Autodesk Fusion 360 part; units mm, degrees
note: some values were not read from the file. Chosen so that the rebuilt part matches the saved one: which pieces of a blend or face edit are solid. Set by a fixed rule: which sketch regions a step uses.
(part 2 of 2)
  line L392 (-39.9447, 99.1082) -> (-40.4511, 101.9789)
  line L393 (-40.4511, 101.9789) -> (-40.8173, 104.0543)
  line L394 (-40.8173, 104.0543) -> (-41.1737, 106.0754)
  line L395 (-41.1737, 106.0754) -> (-42.1677, 111.7124)
  line L396 (-42.1677, 111.7124) -> (-51.7977, 110.0143)
  line L397 (-51.7977, 110.0143) -> (-57.5307, 109.0036)
  line L398 (-57.5307, 109.0036) -> (-57.0143, 106.0757)
  line L399 (-57.0143, 106.0757) -> (-56.9434, 105.6722)
  line L400 (-22.1028, 107.3526) -> (-22.6759, 110.6014)
  line L401 (-22.6759, 110.6014) -> (-23.3222, 114.2669)
  line L402 (-23.3222, 114.2669) -> (-24.0445, 118.3627)
  line L403 (-24.0445, 118.3627) -> (-24.3258, 119.9557)
  line L404 (-24.3258, 119.9557) -> (-27.2217, 119.4446)
  line L405 (-27.2217, 119.4446) -> (-35.4137, 118.0002)
  line L406 (-35.4137, 118.0002) -> (-39.6875, 117.2461)
  line L407 (-39.6875, 117.2461) -> (-39.1623, 114.2664)
  line L408 (-39.1623, 114.2664) -> (-38.816, 112.3021)
  line L409 (-38.816, 112.3021) -> (-37.7177, 106.0746)
  line L410 (-37.7177, 106.0746) -> (-37.4658, 104.6443)
  line L411 (-37.4658, 104.6443) -> (-35.4137, 105.006)
  line L412 (-35.4137, 105.006) -> (-29.3531, 106.0746)
  line L413 (-29.3531, 106.0746) -> (-22.1028, 107.3526)
  line L414 (-85.4379, 28.9057) -> (-100.801, 26.198)
  line L415 (-100.801, 26.198) -> (-98.9954, 15.9628)
  line L416 (-98.9954, 15.9628) -> (-98.5779, 13.5969)
  line L417 (-98.5779, 13.5969) -> (-85.1554, 15.9628)
  line L418 (-85.1554, 15.9628) -> (-84.5661, 16.0668)
  line L419 (-84.5661, 16.0668) -> (-83.2149, 16.3049)
  line L420 (-83.2149, 16.3049) -> (-84.5661, 23.9628)
  line L421 (-84.5661, 23.9628) -> (-85.4379, 28.9057)
  line L422 (-105.1938, 50.9886) -> (-100.9499, 51.7366)
  line L423 (-100.9499, 51.7366) -> (-92.7579, 53.1807)
  line L424 (-92.7579, 53.1807) -> (-89.8308, 53.6967)
  line L425 (-89.8308, 53.6967) -> (-90.3997, 56.9225)
  line L426 (-90.3997, 56.9225) -> (-91.8451, 65.1145)
  line L427 (-91.8451, 65.1145) -> (-92.0538, 66.2977)
  line L428 (-92.0538, 66.2977) -> (-92.7576, 66.1736)
  line L429 (-92.7576, 66.1736) -> (-98.7671, 65.1145)
  line L430 (-98.7671, 65.1145) -> (-100.9497, 64.73)
  line L431 (-100.9497, 64.73) -> (-107.4155, 63.5905)
  line L432 (-107.4155, 63.5905) -> (-107.4018, 63.513)
  line L433 (-107.4018, 63.513) -> (-106.2397, 56.9225)
  line L434 (-106.2397, 56.9225) -> (-105.1938, 50.9886)
  line L435 (-47.6311, 52.8267) -> (-46.9085, 48.731)
  line L436 (-46.9085, 48.731) -> (-46.5989, 46.976)
  line L437 (-46.5989, 46.976) -> (-45.4636, 40.5389)
  line L438 (-45.4636, 40.5389) -> (-45.4099, 40.2339)
  line L439 (-45.4099, 40.2339) -> (-43.6795, 40.5389)
  line L440 (-43.6795, 40.5389) -> (-35.4139, 41.996)
  line L441 (-35.4139, 41.996) -> (-30.0471, 42.9419)
  line L442 (-30.0471, 42.9419) -> (-31.0682, 48.731)
  line L443 (-31.0682, 48.731) -> (-32.2699, 55.545)
  line L444 (-32.2699, 55.545) -> (-35.4139, 54.9907)
  line L445 (-35.4139, 54.9907) -> (-43.606, 53.5466)
  line L446 (-43.606, 53.5466) -> (-47.6332, 52.8368)
  line L447 (-47.6332, 52.8368) -> (-47.6311, 52.8267)
  line L448 (-44.1788, 34.1749) -> (-43.856, 32.3469)
  line L449 (-43.856, 32.3469) -> (-42.4101, 24.1549)
  line L450 (-42.4101, 24.1549) -> (-41.9545, 21.5739)
  line L451 (-41.9545, 21.5739) -> (-35.4134, 22.7267)
  line L452 (-35.4134, 22.7267) -> (-27.3129, 24.1546)
  line L453 (-27.3129, 24.1546) -> (-26.5925, 24.2813)
  line L454 (-26.5925, 24.2813) -> (-28.0151, 32.3464)
  line L455 (-28.0151, 32.3464) -> (-28.8152, 36.8832)
  line L456 (-28.8152, 36.8832) -> (-35.4134, 35.7198)
  line L457 (-35.4134, 35.7198) -> (-43.6055, 34.2754)
  line L458 (-43.6055, 34.2754) -> (-44.1788, 34.1749)
  line L459 (-76.3738, 14.4656) -> (-68.1818, 15.9097)
  line L460 (-68.1818, 15.9097) -> (-67.881, 15.9626)
  line L461 (-67.881, 15.9626) -> (-63.9839, 16.6497)
  line L462 (-63.9839, 16.6497) -> (-65.3079, 24.1546)
  line L463 (-65.3079, 24.1546) -> (-66.0299, 28.2506)
  line L464 (-66.0299, 28.2506) -> (-66.2067, 29.2515)
  line L465 (-66.2067, 29.2515) -> (-68.1818, 28.9033)
  line L466 (-68.1818, 28.9033) -> (-81.57, 26.5435)
  line L467 (-81.57, 26.5435) -> (-79.7026, 15.9626)
  line L468 (-79.7026, 15.9626) -> (-79.3459, 13.9414)
  line L469 (-79.3459, 13.9414) -> (-76.3738, 14.4656)
  line L470 (-17.1048, 98.5898) -> (-2.6458, 101.138)
  line L471 (-2.6458, 101.138) -> (-1.7428, 101.2973)
  line L472 (-1.7428, 101.2973) -> (-2.6458, 106.4194)
  line L473 (-2.6458, 106.4194) -> (-3.9648, 113.901)
  line L474 (-3.9648, 113.901) -> (-19.0296, 111.2443)
  line L475 (-19.0296, 111.2443) -> (-19.3275, 111.1922)
  line L476 (-19.3275, 111.1922) -> (-19.0296, 109.5023)
  line L477 (-19.0296, 109.5023) -> (-17.1048, 98.5898)
  line L478 (-27.2217, 48.5214) -> (-26.035, 48.7307)
  line L479 (-26.035, 48.7307) -> (-19.0296, 49.966)
  line L480 (-19.0296, 49.966) -> (-12.1245, 51.1839)
  line L481 (-12.1245, 51.1839) -> (-13.1366, 56.9227)
  line L482 (-13.1366, 56.9227) -> (-14.3465, 63.7855)
  line L483 (-14.3465, 63.7855) -> (-19.0294, 62.9603)
  line L484 (-19.0294, 62.9603) -> (-27.2214, 61.5162)
  line L485 (-27.2214, 61.5162) -> (-29.7093, 61.0777)
  line L486 (-29.7093, 61.0777) -> (-29.699, 61.0187)
  line L487 (-29.699, 61.0187) -> (-28.9766, 56.9227)
  line L488 (-28.9766, 56.9227) -> (-27.5315, 48.7307)
  line L489 (-27.5315, 48.7307) -> (-27.4865, 48.4746)
  line L490 (-27.4865, 48.4746) -> (-27.2217, 48.5214)
  line L491 (-59.7657, 12.3216) -> (-51.7977, 13.7266)
  line L492 (-51.7977, 13.7266) -> (-44.4037, 15.0299)
  line L493 (-44.4037, 15.0299) -> (-44.5685, 15.9628)
  line L494 (-44.5685, 15.9628) -> (-46.0134, 24.1549)
  line L495 (-46.0134, 24.1549) -> (-46.6267, 27.632)
  line L496 (-46.6267, 27.632) -> (-51.7977, 26.7203)
  line L497 (-51.7977, 26.7203) -> (-59.9898, 25.2756)
  line L498 (-59.9898, 25.2756) -> (-61.9898, 24.9232)
  line L499 (-61.9898, 24.9232) -> (-61.8543, 24.1551)
  line L500 (-61.8543, 24.1551) -> (-60.4083, 15.9631)
  line L501 (-60.4083, 15.9631) -> (-59.9898, 13.5911)
  line L502 (-59.9898, 13.5911) -> (-59.7657, 12.3216)
  line L503 (-117.334, 10.2986) -> (-109.1417, 11.7422)
  line L504 (-109.1417, 11.7422) -> (-108.4355, 11.8668)
  line L505 (-108.4355, 11.8668) -> (-102.0228, 12.9969)
  line L506 (-102.0228, 12.9969) -> (-102.5459, 15.9628)
  line L507 (-102.5459, 15.9628) -> (-103.9902, 24.1549)
  line L508 (-103.9902, 24.1549) -> (-104.2448, 25.599)
  line L509 (-104.2448, 25.599) -> (-109.1419, 24.7356)
  line L510 (-109.1419, 24.7356) -> (-112.4368, 24.1549)
  line L511 (-112.4368, 24.1549) -> (-117.3342, 23.2915)
  line L512 (-117.3342, 23.2915) -> (-119.6081, 22.8907)
  line L513 (-119.6081, 22.8907) -> (-118.386, 15.9626)
  line L514 (-118.386, 15.9626) -> (-117.385, 10.2896)
  line L515 (-117.385, 10.2896) -> (-117.334, 10.2986)
  line L516 (-72.925, 87.1937) -> (-68.1818, 88.0298)
  line L517 (-68.1818, 88.0298) -> (-58.7589, 89.6906)
  line L518 (-58.7589, 89.6906) -> (-57.562, 89.902)
  line L519 (-57.562, 89.902) -> (-58.2472, 93.7866)
  line L520 (-58.2472, 93.7866) -> (-58.9695, 97.8829)
  line L521 (-58.9695, 97.8829) -> (-59.7847, 102.5059)
  line L522 (-59.7847, 102.5059) -> (-68.1818, 101.0259)
  line L523 (-68.1818, 101.0259) -> (-75.1478, 99.7974)
  line L524 (-75.1478, 99.7974) -> (-74.8101, 97.8829)
  line L525 (-74.8101, 97.8829) -> (-73.3653, 89.6906)
  line L526 (-73.3653, 89.6906) -> (-72.925, 87.1937)
  line L527 (-84.5661, 90.283) -> (-77.1416, 91.5919)
  line L528 (-77.1416, 91.5919) -> (-78.2505, 97.8829)
  line L529 (-78.2505, 97.8829) -> (-79.3636, 104.1966)
  line L530 (-79.3636, 104.1966) -> (-84.5659, 103.2793)
  line L531 (-84.5659, 103.2793) -> (-94.7266, 101.4868)
  line L532 (-94.7266, 101.4868) -> (-94.0911, 97.8829)
  line L533 (-94.0911, 97.8829) -> (-92.646, 89.6906)
  line L534 (-92.646, 89.6906) -> (-92.5036, 88.8839)
  line L535 (-92.5036, 88.8839) -> (-87.9258, 89.6906)
  line L536 (-87.9258, 89.6906) -> (-84.5661, 90.283)
  line L537 (-117.334, 29.5698) -> (-109.1417, 31.0139)
  line L538 (-109.1417, 31.0139) -> (-105.2335, 31.7029)
  line L539 (-105.2335, 31.7029) -> (-105.3473, 32.3469)
  line L540 (-105.3473, 32.3469) -> (-106.7922, 40.5389)
  line L541 (-106.7922, 40.5389) -> (-107.4568, 44.3058)
  line L542 (-107.4568, 44.3058) -> (-109.1417, 44.0087)
  line L543 (-109.1417, 44.0087) -> (-117.334, 42.5643)
  line L544 (-117.334, 42.5643) -> (-122.8199, 41.597)
  line L545 (-122.8199, 41.597) -> (-122.6331, 40.5389)
  line L546 (-122.6331, 40.5389) -> (-121.1879, 32.3469)
  line L547 (-121.1879, 32.3469) -> (-120.5968, 28.9949)
  line L548 (-120.5968, 28.9949) -> (-117.334, 29.5698)
  line L549 (-89.2709, 70.0887) -> (-84.5661, 70.9187)
  line L550 (-84.5661, 70.9187) -> (-76.3738, 72.363)
  line L551 (-76.3738, 72.363) -> (-73.9079, 72.7977)
  line L552 (-73.9079, 72.7977) -> (-73.9979, 73.3073)
  line L553 (-73.9979, 73.3073) -> (-75.4428, 81.4991)
  line L554 (-75.4428, 81.4991) -> (-75.8899, 84.0354)
  line L555 (-75.8899, 84.0354) -> (-76.1309, 85.4012)
  line L556 (-76.1309, 85.4012) -> (-76.3738, 85.3583)
  line L557 (-76.3738, 85.3583) -> (-84.5661, 83.9134)
  line L558 (-84.5661, 83.9134) -> (-91.4143, 82.7061)
  line L559 (-91.4143, 82.7061) -> (-91.494, 82.6916)
  line L560 (-91.494, 82.6916) -> (-91.2836, 81.4988)
  line L561 (-91.2836, 81.4988) -> (-89.8385, 73.3071)
  line L562 (-89.8385, 73.3071) -> (-89.2709, 70.0887)
  line L563 (-116.8487, 97.8829) -> (-117.3057, 100.4729)
  line L564 (-117.3057, 100.4729) -> (-117.334, 100.4676)
  line L565 (-117.334, 100.4676) -> (-125.5257, 99.0232)
  line L566 (-125.5257, 99.0232) -> (-131.9937, 97.8826)
  line L567 (-131.9937, 97.8826) -> (-132.6687, 97.7633)
  line L568 (-132.6687, 97.7633) -> (-130.4459, 85.1604)
  line L569 (-130.4459, 85.1604) -> (-117.334, 87.4723)
  line L570 (-117.334, 87.4723) -> (-115.0829, 87.8692)
  line L571 (-115.0829, 87.8692) -> (-115.4038, 89.6903)
  line L572 (-115.4038, 89.6903) -> (-116.8487, 97.8829)
  line L573 (-65.2976, 43.6798) -> (-64.7435, 40.5387)
  line L574 (-64.7435, 40.5387) -> (-63.2987, 32.3466)
  line L575 (-63.2987, 32.3466) -> (-63.0746, 31.0756)
  line L576 (-63.0746, 31.0756) -> (-59.9895, 31.6196)
  line L577 (-59.9895, 31.6196) -> (-55.8665, 32.3466)
  line L578 (-55.8665, 32.3466) -> (-51.7975, 33.0642)
  line L579 (-51.7975, 33.0642) -> (-47.7115, 33.7849)
  line L580 (-47.7115, 33.7849) -> (-48.1804, 36.4427)
  line L581 (-48.1804, 36.4427) -> (-48.9027, 40.5387)
  line L582 (-48.9027, 40.5387) -> (-49.9343, 46.3875)
  line L583 (-49.9343, 46.3875) -> (-51.7972, 46.0592)
  line L584 (-51.7972, 46.0592) -> (-65.2976, 43.6798)
  line L585 (-110.7239, 82.346) -> (-110.7107, 82.2711)
  line L586 (-110.7107, 82.2711) -> (-110.5741, 81.4991)
  line L587 (-110.5741, 81.4991) -> (-109.13, 73.3073)
  line L588 (-109.13, 73.3073) -> (-108.5017, 69.7426)
  line L589 (-108.5017, 69.7426) -> (-100.9497, 71.0748)
  line L590 (-100.9497, 71.0748) -> (-93.1386, 72.4519)
  line L591 (-93.1386, 72.4519) -> (-93.2894, 73.307)
  line L592 (-93.2894, 73.307) -> (-94.7343, 81.4988)
  line L593 (-94.7343, 81.4988) -> (-95.3617, 85.0545)
  line L594 (-95.3617, 85.0545) -> (-100.9497, 84.069)
  line L595 (-100.9497, 84.069) -> (-109.1417, 82.6246)
  line L596 (-109.1417, 82.6246) -> (-110.7239, 82.346)
  line L597 (-51.0701, 52.8267) -> (-51.7927, 56.9227)
  line L598 (-51.7927, 56.9227) -> (-51.7977, 56.951)
  line L599 (-51.7977, 56.951) -> (-53.2376, 65.1145)
  line L600 (-53.2376, 65.1145) -> (-53.2429, 65.1423)
  line L601 (-53.2429, 65.1423) -> (-53.2585, 65.1396)
  line L602 (-53.2585, 65.1396) -> (-53.4016, 65.1142)
  line L603 (-53.4016, 65.1142) -> (-68.1818, 62.5078)
  line L604 (-68.1818, 62.5078) -> (-68.6059, 62.4332)
  line L605 (-68.6059, 62.4332) -> (-68.1818, 60.0297)
  line L606 (-68.1818, 60.0297) -> (-66.3826, 49.8322)
  line L607 (-66.3826, 49.8322) -> (-51.7977, 52.4031)
  line L608 (-51.7977, 52.4031) -> (-51.0199, 52.5404)
  line L609 (-51.0199, 52.5404) -> (-51.0701, 52.8267)
  line L610 (-114.0727, 81.6777) -> (-115.0874, 81.4988)
  line L611 (-115.0874, 81.4988) -> (-117.334, 81.1025)
  line L612 (-117.334, 81.1025) -> (-129.4347, 78.9678)
  line L613 (-129.4347, 78.9678) -> (-128.4367, 73.3071)
  line L614 (-128.4367, 73.3071) -> (-127.2127, 66.3649)
  line L615 (-127.2127, 66.3649) -> (-117.334, 68.1069)
  line L616 (-117.334, 68.1069) -> (-111.8494, 69.0737)
  line L617 (-111.8494, 69.0737) -> (-112.5961, 73.3071)
  line L618 (-112.5961, 73.3071) -> (-114.041, 81.4988)
  line L619 (-114.041, 81.4988) -> (-114.0727, 81.6777)
  line L620 (-11.0397, 45.0308) -> (-19.0296, 43.6219)
  line L621 (-19.0296, 43.6219) -> (-26.4014, 42.322)
  line L622 (-26.4014, 42.322) -> (-26.0871, 40.5389)
  line L623 (-26.0871, 40.5389) -> (-25.5442, 37.4608)
  line L624 (-25.5442, 37.4608) -> (-24.642, 32.3469)
  line L625 (-24.642, 32.3469) -> (-24.1787, 29.7209)
  line L626 (-24.1787, 29.7209) -> (-19.0296, 30.6287)
  line L627 (-19.0296, 30.6287) -> (-9.2818, 32.3469)
  line L628 (-9.2818, 32.3469) -> (-8.8164, 32.4292)
  line L629 (-8.8164, 32.4292) -> (-11.0397, 45.0308)
  line L630 (-52.0089, 77.6719) -> (-51.7977, 77.7092)
  line L631 (-51.7977, 77.7092) -> (-43.6057, 79.1541)
  line L632 (-43.6057, 79.1541) -> (-39.51, 79.8769)
  line L633 (-39.51, 79.8769) -> (-36.6458, 80.3817)
  line L634 (-36.6458, 80.3817) -> (-36.843, 81.4991)
  line L635 (-36.843, 81.4991) -> (-38.8689, 92.9841)
  line L636 (-38.8689, 92.9841) -> (-51.7977, 90.7052)
  line L637 (-51.7977, 90.7052) -> (-54.2316, 90.2758)
  line L638 (-54.2316, 90.2758) -> (-54.1285, 89.6908)
  line L639 (-54.1285, 89.6908) -> (-52.6836, 81.4991)
  line L640 (-52.6836, 81.4991) -> (-52.0089, 77.6719)
  line L641 (-15.4329, 69.94) -> (-17.472, 81.4991)
  line L642 (-17.472, 81.4991) -> (-17.6559, 82.541)
  line L643 (-17.6559, 82.541) -> (-19.0296, 82.2992)
  line L644 (-19.0296, 82.2992) -> (-23.5667, 81.4993)
  line L645 (-23.5667, 81.4993) -> (-27.2214, 80.8548)
  line L646 (-27.2214, 80.8548) -> (-33.0174, 79.8332)
  line L647 (-33.0174, 79.8332) -> (-32.5906, 77.4147)
  line L648 (-32.5906, 77.4147) -> (-32.5887, 77.4033)
  line L649 (-32.5887, 77.4033) -> (-32.4734, 76.7495)
  line L650 (-32.4734, 76.7495) -> (-32.2932, 75.7298)
  line L651 (-32.2932, 75.7298) -> (-32.227, 75.3546)
  line L652 (-32.227, 75.3546) -> (-31.8659, 73.3073)
  line L653 (-31.8659, 73.3073) -> (-30.7941, 67.2322)
  line L654 (-30.7941, 67.2322) -> (-19.0291, 69.306)
  line L655 (-19.0291, 69.306) -> (-15.4329, 69.94)
  line L656 (-71.1078, 56.9227) -> (-71.9749, 61.8395)
  line L657 (-71.9749, 61.8395) -> (-72.5533, 65.1148)
  line L658 (-72.5533, 65.1148) -> (-72.8231, 66.644)
  line L659 (-72.8231, 66.644) -> (-76.3738, 66.0178)
  line L660 (-76.3738, 66.0178) -> (-81.497, 65.1148)
  line L661 (-81.497, 65.1148) -> (-84.5661, 64.5737)
  line L662 (-84.5661, 64.5737) -> (-88.1859, 63.9358)
  line L663 (-88.1859, 63.9358) -> (-86.9487, 56.9227)
  line L664 (-86.9487, 56.9227) -> (-86.2264, 52.8267)
  line L665 (-86.2264, 52.8267) -> (-85.9631, 51.3347)
  line L666 (-85.9631, 51.3347) -> (-84.5664, 51.581)
  line L667 (-84.5664, 51.581) -> (-70.6004, 54.0427)
  line L668 (-70.6004, 54.0427) -> (-71.1078, 56.9227)
  line L669 (-110.7649, 62.9206) -> (-117.334, 61.7627)
  line L670 (-117.334, 61.7627) -> (-125.5257, 60.3189)
  line L671 (-125.5257, 60.3189) -> (-126.1277, 60.2128)
  line L672 (-126.1277, 60.2128) -> (-125.5474, 56.9227)
  line L673 (-125.5474, 56.9227) -> (-124.1026, 48.7307)
  line L674 (-124.1026, 48.7307) -> (-123.9046, 47.6107)
  line L675 (-123.9046, 47.6107) -> (-123.8814, 47.6149)
  line L676 (-123.8814, 47.6149) -> (-117.5531, 48.731)
  line L677 (-117.5531, 48.731) -> (-117.334, 48.7696)
  line L678 (-117.334, 48.7696) -> (-108.5419, 50.3198)
  line L679 (-108.5419, 50.3198) -> (-109.7068, 56.9227)
  line L680 (-109.7068, 56.9227) -> (-110.7649, 62.9206)
  line L681 (-50.8616, 71.5666) -> (-49.7234, 65.1148)
  line L682 (-49.7234, 65.1148) -> (-48.6386, 58.9658)
  line L683 (-48.6386, 58.9658) -> (-35.4137, 61.2979)
  line L684 (-35.4137, 61.2979) -> (-33.2766, 61.6746)
  line L685 (-33.2766, 61.6746) -> (-33.8831, 65.1148)
  line L686 (-33.8831, 65.1148) -> (-35.3269, 73.307)
  line L687 (-35.3269, 73.307) -> (-35.4137, 73.7989)
  line L688 (-35.4137, 73.7989) -> (-35.4976, 74.2754)
  line L689 (-35.4976, 74.2754) -> (-39.5097, 73.5685)
  line L690 (-39.5097, 73.5685) -> (-40.9932, 73.307)
  line L691 (-40.9932, 73.307) -> (-50.8616, 71.5666)
  circle A2 centre (-9.2275, 58.7363) radius 1.1
  circle A3 centre (-44.1849, 9.3587) radius 1.1
  circle A4 centre (-19.4818, 116.8758) radius 1.1
  circle A5 centre (-35.5447, 77.4392) radius 1.1
  circle A6 centre (-61.567, 107.9028) radius 1.1
  circle A7 centre (-85.9131, 48.171) radius 1.1
  circle A8 centre (-132.9571, 103.4239) radius 1.1
  circle A9 centre (-101.7651, 7.3328) radius 1.1
  dimension "d14" = 2.2
  dimension "d16" = 2.2
  dimension "d18" = 2.2
  dimension "d20" = 2.2
  dimension "d22" = 2.2
  dimension "d24" = 2.2
  dimension "d26" = 2.2
  dimension "d28" = 2.2
  measures "d14" diameter of A2
  measures "d16" diameter of A3
  measures "d18" diameter of A4
  measures "d20" diameter of A5
  measures "d22" diameter of A6
  measures "d24" diameter of A7
  measures "d26" diameter of A8
  measures "d28" diameter of A9
extrude "Extrude5" cut sketch "Sketch5" against normal blind 5 contours A2 | A3 | A4 | A5 | A6 | A7 | A8 | A9 bodies 1
sketch "Sketch6" plane through (0, 0, -6.1587) normal (0, 0, -1) x (-1, 0, 0)
  line L0 (-123.7575, 0) -> (12.0737, 0)
  line L1 (12.0737, 0) -> (12.0737, 16.7)
  line L2 (12.0737, 16.7) -> (-123.7575, 16.7)
  line L3 (-123.7575, 16.7) -> (-123.7575, 0)
  line L4 (-8.3443, 16.406) -> (-16.8443, 16.406)
  line L5 (-17.8443, 15.406) -> (-17.8443, 3.406)
  line L6 (-16.8443, 2.406) -> (-8.3443, 2.406)
  line L7 (-7.3443, 3.406) -> (-7.3443, 15.406)
  arc A0 (-16.8443, 16.406) -> (-17.8443, 15.406) centre (-16.8443, 15.406) ccw
  arc A1 (-7.3443, 15.406) -> (-8.3443, 16.406) centre (-8.3443, 15.406) ccw
  arc A2 (-17.8443, 3.406) -> (-16.8443, 2.406) centre (-16.8443, 3.406) ccw
  arc A3 (-8.3443, 2.406) -> (-7.3443, 3.406) centre (-8.3443, 3.406) ccw
  line L8 (-15.9913, 14.35) -> (-9.1913, 14.35)
  line L9 (-8.5913, 13.75) -> (-8.5913, 11.85)
  line L10 (-9.1913, 11.25) -> (-15.9913, 11.25)
  line L11 (-16.5913, 11.85) -> (-16.5913, 13.75)
  arc A4 (-15.9913, 14.35) -> (-16.5913, 13.75) centre (-15.9913, 13.75) ccw
  arc A5 (-8.5913, 13.75) -> (-9.1913, 14.35) centre (-9.1913, 13.75) ccw
  arc A6 (-9.1913, 11.25) -> (-8.5913, 11.85) centre (-9.1913, 11.85) ccw
  arc A7 (-16.5913, 11.85) -> (-15.9913, 11.25) centre (-15.9913, 11.85) ccw
  line L12 (-16.0111, 4.463) -> (-9.2111, 4.463)
  line L13 (-8.6111, 5.063) -> (-8.6111, 6.963)
  line L14 (-9.2111, 7.563) -> (-16.0111, 7.563)
  line L15 (-16.6111, 6.963) -> (-16.6111, 5.063)
  arc A8 (-16.0111, 7.563) -> (-16.6111, 6.963) centre (-16.0111, 6.963) ccw
  arc A9 (-8.6111, 6.963) -> (-9.2111, 7.563) centre (-9.2111, 6.963) ccw
  arc A10 (-9.2111, 4.463) -> (-8.6111, 5.063) centre (-9.2111, 5.063) ccw
  arc A11 (-16.6111, 5.063) -> (-16.0111, 4.463) centre (-16.0111, 5.063) ccw
  point P0 (-7.3443, 16.406)
  point P1 (-17.8443, 16.406)
  point P2 (-7.3443, 2.406)
  point P3 (-16.5913, 14.35)
  point P4 (-8.5913, 14.35)
  point P5 (-16.5913, 11.25)
  point P6 (-16.6111, 4.463)
  point P7 (-8.6111, 4.463)
  point P8 (-16.6111, 7.563)
  dimension "d33" = 10.5
  dimension "d34" = 14
  dimension "d35" = 1
  dimension "d36" = 1
  dimension "d37" = 1
  dimension "d38" = 1
  dimension "d46" = 8
  dimension "d47" = 3.1
  dimension "d48" = 0.6
  dimension "d49" = 0.6
  dimension "d52" = 3.1
  dimension "d53" = 8
  dimension "d54" = 0.6
  measures "d33" distance of P0 P1
  measures "d34" distance of P0 P2
  measures "d35" radius of A0
  measures "d36" radius of A1
  measures "d37" radius of A2
  measures "d38" radius of A3
  measures "d46" distance of P3 P4
  measures "d47" distance of P3 P5
  measures "d48" radius of A4
  measures "d49" radius of A5
  measures "d52" distance of P6 P8
  measures "d53" distance of P6 P7
  measures "d54" radius of A8
extrude "Extrude6" cut sketch "Sketch6" against normal blind 2.25 contours L4 L5 L6 L7 A0 A1 A2 A3 bodies 1
extrude "Extrude7" cut 2 faces at (11.4579, 13.3167, -6.1587) (11.4778, 6.5297, -6.1587) along direction (0, 0, 1) blind 4 on bodies 1 bodies 1
sketch "Sketch7" plane through (0, 0, 0) normal (0, -1, 0) x (1, 0, 0)
  circle A0 centre (85.9131, 48.171) radius 1.1
  circle A1 centre (19.4818, 116.8758) radius 1.1
  circle A2 centre (35.5447, 77.4392) radius 1.1
  circle A3 centre (44.1849, 9.3587) radius 1.1
  circle A4 centre (132.9571, 103.4239) radius 1.1
  circle A5 centre (9.2275, 58.7363) radius 1.1
  circle A6 centre (61.567, 107.9028) radius 1.1
  circle A7 centre (101.7651, 7.3328) radius 1.1
  line L0 (-12.0737, -6.1587) -> (123.7575, -6.1587)
  line L1 (123.7575, -6.1587) -> (124.5415, -6.0984)
  line L2 (124.5415, -6.0984) -> (125.312, -5.9396)
  line L3 (125.312, -5.9396) -> (125.3112, -5.9396)
  line L4 (125.3112, -5.9396) -> (126.0554, -5.6864)
  line L5 (126.0554, -5.6864) -> (126.7632, -5.3411)
  line L6 (126.7632, -5.3411) -> (127.4204, -4.9101)
  line L7 (127.4204, -4.9101) -> (128.0208, -4.4006)
  line L8 (128.0208, -4.4006) -> (128.0213, -4.4006)
  line L9 (128.0213, -4.4006) -> (128.5505, -3.8201)
  line L10 (128.5505, -3.8201) -> (129.004, -3.1771)
  line L11 (129.004, -3.1771) -> (129.3736, -2.4831)
  line L12 (129.3736, -2.4831) -> (129.6532, -1.7473)
  line L13 (129.6532, -1.7473) -> (129.8382, -0.9829)
  line L14 (129.8382, -0.9829) -> (148.3492, 103.9992)
  line L15 (148.3492, 103.9992) -> (148.4371, 104.7803)
  line L16 (148.4371, 104.7803) -> (148.4363, 104.7795)
  line L17 (148.4363, 104.7795) -> (148.4249, 105.5666)
  line L18 (148.4249, 105.5666) -> (148.4257, 105.5672)
  line L19 (148.4257, 105.5672) -> (148.3154, 106.3461)
  line L20 (148.3154, 106.3461) -> (148.3154, 106.3448)
  line L21 (148.3154, 106.3448) -> (148.1098, 107.1036)
  line L22 (148.1098, 107.1036) -> (147.8108, 107.8315)
  line L23 (147.8108, 107.8315) -> (147.4213, 108.5146)
  line L24 (147.4213, 108.5146) -> (146.9501, 109.1449)
  line L25 (146.9501, 109.1449) -> (146.9488, 109.1457)
  line L26 (146.9488, 109.1457) -> (146.4043, 109.7113)
  line L27 (146.4043, 109.7113) -> (146.4043, 109.7103)
  line L28 (146.4043, 109.7103) -> (145.7907, 110.204)
  line L29 (145.7907, 110.204) -> (145.7907, 110.2045)
  line L30 (145.7907, 110.2045) -> (145.121, 110.6167)
  line L31 (145.121, 110.6167) -> (145.121, 110.6159)
  line L32 (145.121, 110.6159) -> (144.4046, 110.9403)
  line L33 (144.4046, 110.9403) -> (143.6531, 111.1734)
  line L34 (143.6531, 111.1734) -> (19.6824, 136.2139)
  line L35 (19.6824, 136.2139) -> (18.9079, 136.3501)
  line L36 (18.9079, 136.3501) -> (18.9079, 136.3493)
  line L37 (18.9079, 136.3493) -> (18.1216, 136.3877)
  line L38 (18.1216, 136.3877) -> (-12.0737, 136.3885)
  line L39 (-12.0737, 136.3885) -> (-12.0737, -6.1587)
  line L40 (18.2694, 118.9758) -> (17.0569, 116.8758)
  line L41 (17.0569, 116.8758) -> (18.2694, 114.7758)
  line L42 (18.2694, 114.7758) -> (20.6942, 114.7758)
  line L43 (20.6942, 114.7758) -> (21.9067, 116.8758)
  line L44 (21.9067, 116.8758) -> (20.6942, 118.9758)
  line L45 (20.6942, 118.9758) -> (18.2694, 118.9758)
  line L46 (34.3322, 79.5392) -> (33.1198, 77.4392)
  line L47 (33.1198, 77.4392) -> (34.3322, 75.3392)
  line L48 (34.3322, 75.3392) -> (36.7571, 75.3392)
  line L49 (36.7571, 75.3392) -> (37.9695, 77.4392)
  line L50 (37.9695, 77.4392) -> (36.7571, 79.5392)
  line L51 (36.7571, 79.5392) -> (34.3322, 79.5392)
  line L52 (8.015, 60.8363) -> (6.8026, 58.7363)
  line L53 (6.8026, 58.7363) -> (8.015, 56.6363)
  line L54 (8.015, 56.6363) -> (10.4399, 56.6363)
  line L55 (10.4399, 56.6363) -> (11.6523, 58.7363)
  line L56 (11.6523, 58.7363) -> (10.4399, 60.8363)
  line L57 (10.4399, 60.8363) -> (8.015, 60.8363)
  line L58 (60.3545, 110.0028) -> (59.1421, 107.9028)
  line L59 (59.1421, 107.9028) -> (60.3545, 105.8028)
  line L60 (60.3545, 105.8028) -> (62.7794, 105.8028)
  line L61 (62.7794, 105.8028) -> (63.9918, 107.9028)
  line L62 (63.9918, 107.9028) -> (62.7794, 110.0028)
  line L63 (62.7794, 110.0028) -> (60.3545, 110.0028)
  line L64 (131.7447, 105.5239) -> (130.5322, 103.4239)
  line L65 (130.5322, 103.4239) -> (131.7447, 101.3239)
  line L66 (131.7447, 101.3239) -> (134.1695, 101.3239)
  line L67 (134.1695, 101.3239) -> (135.382, 103.4239)
  line L68 (135.382, 103.4239) -> (134.1695, 105.5239)
  line L69 (134.1695, 105.5239) -> (131.7447, 105.5239)
  line L70 (84.7007, 50.271) -> (83.4882, 48.171)
  line L71 (83.4882, 48.171) -> (84.7007, 46.071)
  line L72 (84.7007, 46.071) -> (87.1256, 46.071)
  line L73 (87.1256, 46.071) -> (88.338, 48.171)
  line L74 (88.338, 48.171) -> (87.1256, 50.271)
  line L75 (87.1256, 50.271) -> (84.7007, 50.271)
  line L76 (42.9725, 11.4587) -> (41.76, 9.3587)
  line L77 (41.76, 9.3587) -> (42.9725, 7.2587)
  line L78 (42.9725, 7.2587) -> (45.3973, 7.2587)
  line L79 (45.3973, 7.2587) -> (46.6098, 9.3587)
  line L80 (46.6098, 9.3587) -> (45.3973, 11.4587)
  line L81 (45.3973, 11.4587) -> (42.9725, 11.4587)
  line L82 (100.5527, 9.4328) -> (99.3402, 7.3328)
  line L83 (99.3402, 7.3328) -> (100.5527, 5.2328)
  line L84 (100.5527, 5.2328) -> (102.9775, 5.2328)
  line L85 (102.9775, 5.2328) -> (104.19, 7.3328)
  line L86 (104.19, 7.3328) -> (102.9775, 9.4328)
  line L87 (102.9775, 9.4328) -> (100.5527, 9.4328)
  point P0 (19.4818, 116.8758)
  point P1 (35.5447, 77.4392)
  point P2 (9.2275, 58.7363)
  point P3 (61.567, 107.9028)
  point P4 (132.9571, 103.4239)
  point P5 (85.9131, 48.171)
  point P6 (44.1849, 9.3587)
  point P7 (101.7651, 7.3328)
move_face "OffsetFaces1" offset 1.15 1 faces at (15.285, 1.3333, 0.0568) on bodies 1
move_face "OffsetFaces2" offset 1.15 1 faces at (-0.1293, 1.3333, 0.114) on bodies 1
extrude "Extrude8" cut sketch "Sketch7" against normal blind 2.2 contours L40 L41 L42 L43 L44 L45 | L46 L47 L48 L49 L50 L51 | L52 L53 L54 L55 L56 L57 | L58 L59 L60 L61 L62 L63 | L64 L65 L66 L67 L68 L69 | L70 L71 L72 L73 L74 L75 | L76 L77 L78 L79 L80 L81 | L82 L83 L84 L85 L86 L87 bodies 1
ref_plane "WorkPlane1" through (-22.0737, 8.35, 65.1149) normal (-1, 0, 0) x (0, 0, 1)
mirror "Mirror1" about plane through (-22.0737, 8.35, 65.1149) normal (-1, 0, 0) of bodies 1 makes body 2
mirror "Mirror2" about plane through (-22.0737, 8.35, 65.1149) normal (-1, 0, 0) of bodies 2 makes body 3
hidden bodies 1
